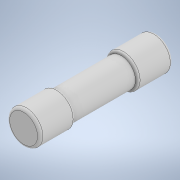
# Autodesk Inventor part: Fusible de 2A
Saved by Autodesk Inventor 2021 (Build 250183000, 183)
## iProperties
Created: 2021-05-26
Part Number: Fusible de 2A
Material: Generic
Document SubType Name: Modeling
Designer: Nelson
Density: 29.1718 g/cm^3
Appearance: Default
Mass: 10 g
Surface Area: 3.32619 cm^2
Volume: 0.342797 cm^3
Author: Nelson
Autodesk Inventor part; units mm, degrees
ref_plane "YZ Plane" through (0, 0, 0) normal (1, 0, 0) x (0, 1, 0)
ref_plane "XZ Plane" through (0, 0, 0) normal (0, 1, 0) x (-1, 0, 0)
ref_plane "XY Plane" through (0, 0, 0) normal (0, 0, 1) x (1, 0, 0)
sketch "Sketch2" plane through (0, 0, 0) normal (1, 0, 0) x (0, 1, 0)
  line L0 (0, 0) -> (2.5, 0)
  line L1 (2.5, 0) -> (2.5, -5.3)
  line L2 (2.5, -5.3) -> (2.15, -5.3)
  line L3 (2.15, -5.3) -> (2.15, -14.7)
  line L4 (2.15, -14.7) -> (2.5, -14.7)
  line L5 (2.5, -14.7) -> (2.5, -20)
  line L6 (2.5, -20) -> (0, -20)
  line L7 (0, -20) -> (0, 0)
  dimension "d1" = 2.5
  dimension "d2" = 5.3
  dimension "d3" = 0.35
  dimension "d4" = 9.4
  dimension "d5" = 0.35
  dimension "d6" = 5.3
  dimension "d7" = 2.5
  constraints: 16 end point, 3 perpendicular, 2 point on line, 1 horizontal, 1 vertical
  measures "d1" distance of L0.start L0.end
  measures "d2" distance of L0.end L1.end
  measures "d3" distance of L1.end L2.end
  measures "d4" distance of L2.end L3.end
  measures "d5" distance of L3.end L4.end
  measures "d6" distance of L4.end L5.end
  measures "d7" distance of L5.end L6.end
revolve "Revolution1" add sketch "Sketch2" angle 360 about axis through (0, 0, -20) along (0, 0, 1)
fillet "Fillet4" radius 0.4 2 edges at (0, -2.5, -20) (0, -2.5, 0)
fillet "Fillet5" radius 0.35 2 edges at (0, -2.5, -14.7) (0, -2.5, -5.3)
equation "\"d5\" = d3"
equation "\"d6\" = d2"
equation "\"d7\" = d1"
body "Solid1"
